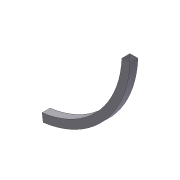
# Autodesk Inventor part: Shooter_Frame_RearGuide
Saved by Autodesk Inventor 2012 (Build 160160000, 160)
## iProperties
Created: 2012-01-18
Part Number: Shooter_Frame_RearGuide
Material: Aluminum-6061
Document SubType Name: Modeling
Designer: JesseK
Mass: 174.62 g
Surface Area: 814.81 cm^2
Volume: 64.4354 cm^3
Density: 2.71 g/cm^3
Author: JesseK
Autodesk Inventor part; units mm, degrees
ref_plane "YZ Plane" through (0, 0, 0) normal (1, 0, 0) x (0, 1, 0)
ref_plane "XZ Plane" through (0, 0, 0) normal (0, 1, 0) x (-1, 0, 0)
ref_plane "XY Plane" through (0, 0, 0) normal (0, 0, 1) x (1, 0, 0)
sketch "Sketch1" plane through (0, 0, 0) normal (0, 0, 1) x (1, 0, 0)
  arc A0 (38.1676, -289.5957) -> (291.8238, -12.7) centre (0, 0) ccw
  arc A1 (41.4865, -314.7779) -> (317.2459, -12.7) centre (0, 0) ccw
  line L0 (38.1676, -289.5957) -> (41.4865, -314.7779)
  line L1 (291.8238, -12.7) -> (317.2459, -12.7)
  line L2 (0, 0) -> (38.1676, -289.5957) construction
  line L3 (0, -292.1) -> (0, 0) construction
  line L4 (291.8238, -12.7) -> (0, 0) construction
  line L5 (291.8238, 0) -> (317.2459, 0) construction
  line L6 (317.2459, 0) -> (317.2459, -12.7) construction
  line L7 (317.2459, -12.7) -> (291.8238, -12.7) construction
  line L8 (291.8238, -12.7) -> (291.8238, 0) construction
  line L9 (0, 0) -> (359.7285, 0) construction
  dimension "d0" = 292.1
  dimension "d1" = 25.4
  dimension "d9" = 12.7
  dimension "d10" = 80
  constraints: 21 end point, 4 point on circle, 3 coincident, 2 centre point, 2 horizontal, 2 parallel, 1 collinear, 1 perpendicular, 1 point on line, 1 vertical
  measures "d0" radius of A0
  measures "d1" radial gap between concentric circles of A1 A0
  measures "d9" distance of L1.start L5.start
  measures "d10" angle of L2 L4
extrude "Extrusion1" add sketch "Sketch1" along normal blind 25.4
shell "Shell1" thickness 1.5875 removed faces 2 at (300.2978, -12.7, 8.4667) at (40.3802, -306.3838, 8.4667)
body "Solid1"
